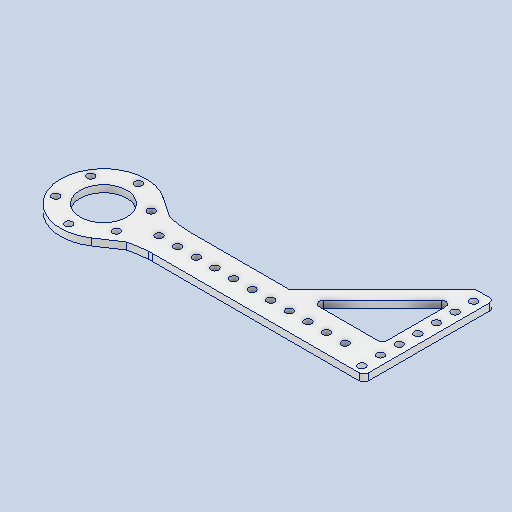
# Autodesk Inventor part: climber-arm-brace
Saved by Autodesk Inventor 2025.2 (Build 292293000, 293)
## iProperties
Created: 2025-03-18
Part Number: climber-arm-brace
Material: Aluminum 6061
Document SubType Name: Sheet Metal
Designer: mathe
Density: 2.7 g/cm^3
Sheet Metal Rule: Default
Appearance: Aluminum - Flat
Mass: 91.8837 g
Surface Area: 201.693 cm^2
Volume: 34.031 cm^3
Author: mathe
Autodesk Inventor part; units mm, degrees
ref_plane "YZ Plane" through (0, 0, 0) normal (1, 0, 0) x (0, 1, 0)
ref_plane "XZ Plane" through (0, 0, 0) normal (0, 1, 0) x (-1, 0, 0)
ref_plane "XY Plane" through (0, 0, 0) normal (0, 0, 1) x (1, 0, 0)
sketch "Sketch1" plane through (0, 0, 0) normal (0, 1, 0) x (-1, 0, 0)
  line L0 (-45.818, 12.7) -> (-187.1472, 12.7)
  arc A0 (-187.1472, 12.7) -> (-190.3222, 9.525) centre (-187.1472, 9.525) ccw
  line L1 (-190.3222, 9.525) -> (-190.3222, -73.025)
  arc A1 (-190.3222, -73.025) -> (-187.1472, -76.2) centre (-187.1472, -73.025) ccw
  line L2 (-187.1472, -76.2) -> (-177.6222, -76.2)
  line L3 (-177.6222, -76.2) -> (-114.1222, -12.7)
  line L4 (-114.1222, -12.7) -> (-45.818, -12.7)
  arc A2 (-31.6867, -16.9939) -> (-45.818, -12.7) centre (-45.818, -38.1) ccw
  line L5 (-31.6867, -16.9939) -> (-17.6641, -26.3826)
  arc A3 (-17.6641, -26.3826) -> (-17.6641, 26.3826) centre (0, 0) ccw
  line L6 (-17.6641, 26.3826) -> (-31.6867, 16.9939)
  arc A4 (-45.818, 12.7) -> (-31.6867, 16.9939) centre (-45.818, 38.1) ccw
  line L7 (-174.4472, -12.7) -> (-134.4873, -12.7)
  arc A5 (-132.2423, -18.1201) -> (-134.4873, -12.7) centre (-134.4873, -15.875) ccw
  line L8 (-132.2423, -18.1201) -> (-172.2021, -58.0799)
  arc A6 (-177.6222, -55.8349) -> (-172.2021, -58.0799) centre (-174.4472, -55.8349) ccw
  line L9 (-177.6222, -55.8349) -> (-177.6222, -15.875)
  arc A7 (-174.4472, -12.7) -> (-177.6222, -15.875) centre (-174.4472, -15.875) ccw
  circle A8 centre (-183.9722, 7.62) radius 2.5527
  circle A9 centre (-183.9722, -68.58) radius 2.5527
  circle A10 centre (-183.9722, -55.88) radius 2.5527
  circle A11 centre (-183.9722, -43.18) radius 2.5527
  circle A12 centre (-183.9722, -30.48) radius 2.5527
  circle A13 centre (-183.9722, -17.78) radius 2.5527
  circle A14 centre (-183.9722, -5.08) radius 2.5527
  circle A15 centre (0, 0) radius 12.827
  circle A16 centre (0, -23.8252) radius 2.5527
  circle A17 centre (-20.6332, -11.9126) radius 2.5527
  circle A18 centre (-20.6332, 11.9126) radius 2.5527
  circle A19 centre (0, 23.8252) radius 2.5527
  circle A20 centre (20.6332, 11.9126) radius 2.5527
  circle A21 centre (20.6332, -11.9126) radius 2.5527
  circle A22 centre (-37.9222, 0) radius 2.5527
  circle A23 centre (-50.6222, 0) radius 2.5527
  circle A24 centre (-63.3222, 0) radius 2.5527
  circle A25 centre (-76.0222, 0) radius 2.5527
  circle A26 centre (-88.7222, 0) radius 2.5527
  circle A27 centre (-101.4222, 0) radius 2.5527
  circle A28 centre (-114.1222, 0) radius 2.5527
  circle A29 centre (-126.8222, 0) radius 2.5527
  circle A30 centre (-139.5222, 0) radius 2.5527
  circle A31 centre (-152.2222, 0) radius 2.5527
  circle A32 centre (-164.9222, 0) radius 2.5527
  circle A33 centre (0, 0) radius 15.9131
  arc A34 (-16.251, -24.272) -> (-16.251, 24.272) centre (0, 0) ccw
  line L10 (-16.251, 24.272) -> (-30.2736, 14.8833)
  line L11 (-30.2736, -14.8833) -> (-16.251, -24.272)
  arc A35 (-45.818, 12.7) -> (-30.2736, 14.8833) centre (-48.2316, 86.3103) ccw
  arc A36 (-30.2736, -14.8833) -> (-45.818, -12.7) centre (-48.2316, -86.3103) ccw
  point P0 (-31.6867, -16.9939)
  point P1 (-17.6641, 26.3826)
  point P2 (-114.1222, -12.7)
  point P3 (-132.2423, -18.1201)
  point P4 (-43.2812, -12.827)
  point P5 (-16.251, 24.272)
  point P6 (-43.2812, 12.827)
  dimension "d1" = 31.8262
  dimension "d2" = 2.54
  dimension "d3" = 2.54
  dimension "d4" = 2.54
  measures "d1" diameter of A33
  measures "d2" radial gap between concentric circles of A3 A34
  measures "d3" distance between parallel lines of L6 L10
  measures "d4" distance between parallel lines of L5 L11
extrude "Plate1" add sketch "Sketch1" along normal blind 4.7625 contours A4 A35 L10 A34 L11 A36 A2 L4 L3 L2 A1 L1 A0 L0
equation "\"d0\" = Thickness"
equation "\"BendRadius\" = Thickness"
equation "\"BendReliefWidth\" = Thickness"
equation "\"BendReliefDepth\" = 0.5 * Thickness"
equation "\"CornerReliefSize\" = 4 * Thickness"
equation "\"MinimumRemnant\" = 2 * Thickness"
equation "\"TransitionRadius\" = BendRadius"
equation "\"JacobiRadiusSize\" = BendRadius"
equation "\"GapSize\" = Thickness"
equation "\"Thickness\" = 4.7625"
body "Solid1"
